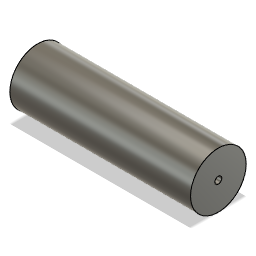
Валы v2 (Autodesk Fusion 360 design; units mm, degrees)
Autodesk Fusion 360 part; units mm, degrees
sketch "Sketch1" plane through (0, 0, 0) normal (1, 0, 0) x (0, 0, -1)
  circle A0 centre (0, 0) radius 20
  circle A1 centre (0, 0) radius 2.5
  dimension "d3" = 5
  constraint coincident A0.centre A1.centre
  constraint concentric A0 A1
  measures "d3" diameter of A1
extrude "Extrude1" add sketch "Sketch1" against normal blind 130
